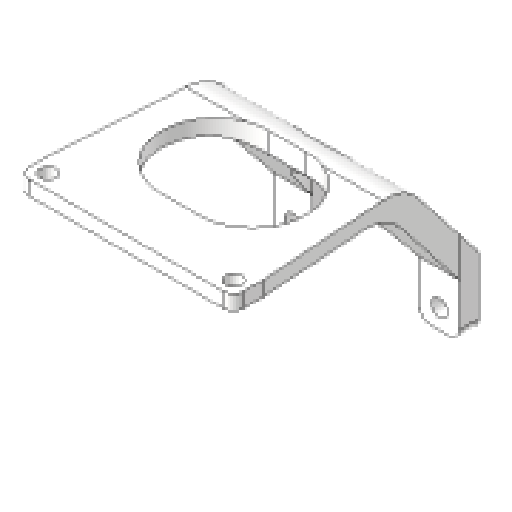
# Autodesk Inventor part: Loading_v1_ABS_EncMount
Saved by Autodesk Inventor 2025.3 (Build 293356000, 356)
## iProperties
Created: 2026-07-06
Part Number: Loading_v1_ABS_EncMount
Material: ABS プラスチック
Document SubType Name: Modeling
Designer: tomoya
Density: 1.06 g/cm^3
Appearance: 滑らか - 白
Author: tomoya
Autodesk Inventor part; units mm, degrees
ref_plane "YZ Plane" through (0, 0, 0) normal (1, 0, 0) x (0, 1, 0)
ref_plane "XY Plane" through (0, 0, 0) normal (0, 0, 1) x (1, 0, 0)
sketch "スケッチ1" plane through (0, 0, 0) normal (0, 0, 1) x (1, 0, 0)
  line L0 (-49.22, 19) -> (-53.22, 19)
  line L1 (-53.22, 19) -> (-53.22, 11)
  line L2 (-53.22, 11) -> (-49.22, 11)
  line L3 (-49.22, 11) -> (-49.22, 19)
  line L4 (-49.22, 19) -> (-6, 22)
  line L5 (-6, 22) -> (0, 22)
  line L6 (0, 22) -> (0, 0)
  line L7 (0, 0) -> (-38.22, 0) construction
  arc A0 (-38.22, 0) -> (-49.22, 11) centre (-49.22, 0) ccw
  line L8 (-49.22, -19) -> (-53.22, -19)
  line L9 (-53.22, -19) -> (-53.22, -11)
  line L10 (-53.22, -11) -> (-49.22, -11)
  line L11 (-49.22, -11) -> (-49.22, -19)
  line L12 (-49.22, -19) -> (-6, -22)
  line L13 (-6, -22) -> (0, -22)
  line L14 (0, -22) -> (0, 0)
  arc A1 (-49.22, -11) -> (-38.22, 0) centre (-49.22, 0) ccw
  line L15 (-6, 22) -> (-6, -22) construction
  line L16 (-22.11, 3.7573) -> (-22.11, -3.7573) construction
  line L17 (-33.22, 3.7573) -> (-33.22, -3.7573)
  line L18 (-11, -3.7573) -> (-11, 3.7573)
  arc A2 (-11, 3.7573) -> (-33.22, 3.7573) centre (-22.11, 3.7573) ccw
  arc A3 (-33.22, -3.7573) -> (-11, -3.7573) centre (-22.11, -3.7573) ccw
  point P0 (-3, 19)
  point P1 (-49.22, 15)
  point P2 (-3, -19)
  point P3 (-22.11, 0)
  point P4 (-22.11, 14.8673)
  point P5 (-33.22, 0)
  point P6 (-6, 0)
  point P7 (-11, 0)
  dimension "d0" = 19
  dimension "d1" = 3
  dimension "d2" = 15
  dimension "d3" = 46.22
  dimension "d4" = 8
  dimension "d5" = 4
  dimension "d6" = 6
  dimension "d7" = 3
  dimension "d8" = 6
  dimension "d9" = 5
  dimension "d10" = 5
  constraints: 40 end point, 9 point on circle, 7 symmetric about line, 5 midpoint, 5 tangent, 4 centre point, 4 perpendicular, 3 horizontal, 3 parallel, 1 line through centre, 1 point on line, 1 other
  measures "d0" vertical distance of L6.end point (-3, 19)
  measures "d1" horizontal distance of L6.end point (-3, 19)
  measures "d2" vertical distance of L6.end point (-49.22, 15)
  measures "d3" distance from line of L3 point (-3, 19)
  measures "d4" distance of L0.end L1.end
  measures "d5" distance of L0.start L0.end
  measures "d6" distance of L4.end L5.end
  measures "d7" distance from line of L5 point (-3, 19)
  measures "d8" distance from line of L4 point (-22.11, 14.867)
  measures "d9" distance of L7.end point (-33.22, 0)
  measures "d10" distance of point (-6, 0) point (-11, 0)
extrude "押し出し1" add sketch "スケッチ1" along normal blind 3
extrude "押し出し2" add sketch "スケッチ1" against normal blind 31 contours L3 L2 L1 L0 | L11 L8 L9 L10
hole "穴1" at (-3, 19, 0) at (-3, -19, 0) direction (0, 0, 1) diameter 3.4 end through all
chamfer "面取り1" distance 16 distance2 20 2 edges at (-49.22, 15, 0) (-49.22, -15, 0) measured on face at (-48.72, -15, 0) measured on face at (-48.72, 15, 0)
chamfer "面取り2" distance 16 distance2 20 2 edges at (-53.22, -15, 3) (-53.22, 15, 3) measured on face at (-52.72, -15, 3) measured on face at (-52.72, 15, 3)
sketch "スケッチ2" plane through (-53.22, 11, -31) normal (-1, 0, 0) x (0, 0, 1)
  line L0 (0, -30) -> (0, -22) projected
  line L1 (0, 0) -> (0, 8) projected
  point P0 (31, -11)
  point P1 (4, 4)
  point P2 (4, -26)
  point P3 (0, -26)
  point P4 (0, 4)
  dimension "d28" = 4
  constraints: 2 horizontal alignment, 2 midpoint, 1 vertical alignment
  measures "d28" distance from line of L1 point (4, 4)
hole "穴2" at (-53.22, 15, -27) at (-53.22, -15, -27) direction (1, 0, 0) diameter 3.4 end through all
fillet "フィレット1" radius 2 4 edges at (-51.22, -19, -31) (-51.22, -11, -31) (-51.22, 11, -31) (-51.22, 19, -31)
fillet "フィレット2" radius 10 2 edges at (-33.22, -11.934, 0) (-33.22, 11.934, 0)
fillet "フィレット3" radius 10 1 edges at (-37.22, 0, 3)
fillet "フィレット4" radius 2 2 edges at (0, -22, 1.5) (0, 22, 1.5)
fillet "フィレット5" radius 2 2 edges at (-53.22, 15, -17) (-53.22, -15, -17)
sketch "スケッチ3" plane through (0, -20, 0) normal (1, 0, 0) x (0, 0, -1)
  line L0 (-3, 0) -> (-3, 40) projected
  line L1 (-3, 13) -> (-2, 13)
  line L2 (-2, 13) -> (-2, 27)
  line L3 (-2, 27) -> (-3, 27)
  point P0 (0, 20)
  point P1 (-2, 20)
  point P2 (-3, 20)
  dimension "d41" = 1
  dimension "d42" = 14
  constraints: 6 end point, 3 perpendicular, 2 midpoint, 2 point on line, 1 horizontal alignment
  measures "d41" distance between parallel lines of L2 L0
  measures "d42" distance of L1.end L2.end
extrude "押し出し3" cut sketch "スケッチ3" against normal through all
ref_plane "作業平面1" through (0, -13, 0) normal (0, 1, 0) x (-1, 0, 0)
ref_plane "作業平面2" through (0, 13, 0) normal (0, 1, 0) x (-1, 0, 0)
sketch "スケッチ5" plane through (0, -13, 0) normal (0, 1, 0) x (-1, 0, 0)
  line L0 (15.9452, 0) -> (0, 0) projected
  line L1 (0, 0) -> (0, 3) projected
  line L2 (0, 3) -> (15.9452, 3) projected
  line L3 (15.9452, 3) -> (15.9452, 0) projected
  line L4 (49.22, -31) -> (49.22, -20) projected
  line L5 (53.22, -17.7016) -> (53.22, -31) projected
  line L6 (49.22, -20) -> (36.2224, -3.753) projected
  arc A0 (36.2224, -3.753) -> (28.4138, 0) centre (28.4138, -10) ccw projected
  line L7 (28.4138, 0) -> (28.2748, 0) projected
  line L8 (28.2748, 0) -> (28.2748, 3) projected
  line L9 (28.2748, 3) -> (32.4138, 3) projected
  arc A1 (40.2224, -0.753) -> (32.4138, 3) centre (32.4138, -7) ccw projected
  line L10 (40.2224, -0.753) -> (52.7817, -16.4522) projected
  arc A2 (53.22, -17.7016) -> (52.7817, -16.4522) centre (51.22, -17.7016) ccw projected
  line L11 (6, 0) -> (6, 3) projected
  line L12 (6, 3) -> (16, 8)
  line L13 (16, 8) -> (33.22, 8)
  line L14 (53.22, -17.7016) -> (53.22, -12)
  arc A3 (53.22, -12) -> (33.22, 8) centre (33.22, -12) ccw
  line L15 (15.9452, 3) -> (28.2748, 3)
  line L16 (53.22, -31) -> (49.22, -31) projected
  line L17 (53.22, -23) -> (56.22, -16)
  line L18 (56.22, -16) -> (56.22, -8.7344)
  line L19 (56.22, -8.7344) -> (48.8374, 0.4939)
  dimension "d47" = 5
  dimension "d48" = 10
  dimension "d49" = 20
  dimension "d54" = 8
  dimension "d55" = 3
  dimension "d56" = 7
  constraints: 14 end point, 3 point on circle, 3 tangent, 2 vertical, 1 centre point, 1 horizontal, 1 parallel, 1 perpendicular, 1 point on line
  measures "d47" distance between parallel lines of L2 L13
  measures "d48" horizontal distance of L11.end L12.end
  measures "d49" radius of A3
  measures "d54" distance from line of L16 L17.start
  measures "d55" distance between parallel lines of L14 L18
  measures "d56" vertical distance of L17.start L17.end
extrude "押し出し4" add sketch "スケッチ5" against normal blind 4 contours L2 L12 L13 A3 L14 A2 L10 A1 L9 L15 | L19 L18 L17 L5 L14 A3
extrude "押し出し5" add sketch "スケッチ5" along normal blind 4 from surface at 26 contours L2 L12 L13 A3 L14 A2 L10 A1 L9 L15 | L19 L18 L17 L5 L14 A3
fillet "フィレット6" radius 10 6 edges at (-56.22, -15, -8.7344) (-56.22, 15, -8.7344) (-56.22, 15, -16) (-56.22, -15, -16) (-16, 15, 8) (-16, -15, 8)
extrude "押し出し6" cut sketch "スケッチ1" along normal through all contours A2 L18 A3 L17
equation "\"d6\" = 2 * d1"
